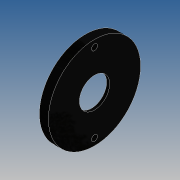
# Autodesk Inventor part: P119PorteLentilleSouple
Saved by Autodesk Inventor 2015 SP1 (Build 190203100, 203)
## iProperties
Created: 2017-01-12
Part Number: P119PorteLentilleSouple
Material: ABS Plastic
Document SubType Name: Modeling
Designer: serge.amoos
Density: 1.06 g/cm^3
Appearance: Smooth - Black
Author: serge.amoos
Autodesk Inventor part; units mm, degrees
ref_plane "YZ Plane" through (0, 0, 0) normal (1, 0, 0) x (0, 1, 0)
ref_plane "XZ Plane" through (0, 0, 0) normal (0, 1, 0) x (-1, 0, 0)
ref_plane "XY Plane" through (0, 0, 0) normal (0, 0, 1) x (1, 0, 0)
sketch "Sketch1" plane through (0, 0, 0) normal (0, 0, 1) x (1, 0, 0)
  line L0 (0, -3.05) -> (0, 18.3) construction
  line L1 (-3.6, 0) -> (0.6, 0) construction
  line L2 (0, 5) -> (0, 15.25)
  line L3 (0, 15.25) -> (-3, 15.25)
  line L4 (-3, 15.25) -> (-3, 11)
  line L5 (-3, 11) -> (-1, 11)
  line L6 (-1, 11) -> (-1, 5)
  line L7 (-1, 5) -> (0, 5)
  point P0 (0, 0)
  dimension "d0" = 30.5
  dimension "d1" = 10
  dimension "d2" = 22
  dimension "d3" = 1
  dimension "d4" = 3
  constraints: 12 end point, 5 perpendicular, 2 point on line
  measures "d0" diameter of L3 L1
  measures "d1" diameter of L6.end L1
  measures "d2" diameter of L5 L1
  measures "d3" distance between parallel lines of L0 L6
  measures "d4" distance between parallel lines of L0 L4
revolve "Revolution1" add sketch "Sketch1" angle 360 about axis through (-10, 0, 0) along (1, 0, 0)
sketch "Sketch2" plane through (-3, 0, 0) normal (-1, 0, 0) x (0, 0, 1)
  line L0 (0, -21.35) -> (0, 21.35) projected
  line L1 (-21.35, 0) -> (21.35, 0) projected
  point P0 (0, 0)
  point P1 (-13, 0)
  dimension "d6" = 13
  constraints: 1 point on line
  measures "d6" distance from line of L0 point (-13, 0)
hole "Hole1" at (-3, 0, -13) direction (1, 0, 0) diameter 2 end through all
mirror "Mirror1" about plane through (0, 0, 0) normal (0, 0, 1) of "Hole1"
body "Solid1"
